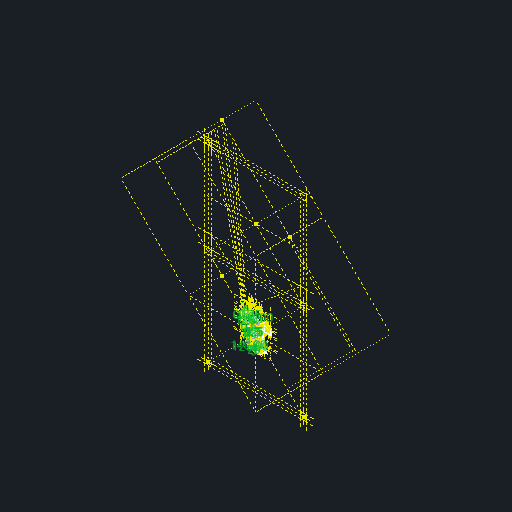
# Autodesk Inventor part: circuit
Saved by Autodesk Inventor 2023.5 (Build 275446000, 446)
## iProperties
Created: 2025-01-11
Part Number: circuit
Material: 一般
Document SubType Name: Modeling
Designer: IshiiLabHonda
Density: 1 g/cm^3
Appearance: 既定
Author: IshiiLabHonda
Autodesk Inventor part; units mm, degrees
ref_plane "YZ Plane" through (0, 0, 0) normal (1, 0, 0) x (0, 1, 0)
ref_plane "XZ Plane" through (0, 0, 0) normal (0, 1, 0) x (-1, 0, 0)
ref_plane "XY Plane" through (0, 0, 0) normal (0, 0, 1) x (1, 0, 0)
derived "chassis.ipt"
sketch "スケッチ1" plane through (0, 0, 0) normal (0, 0, 1) x (1, 0, 0)
  line L0 (0, 0) -> (0, 1) construction
  line L1 (0, 0) -> (1, 0) construction
  line L2 (-90, 90) -> (90, 90) construction
  line L3 (90, 90) -> (90, -90) construction
  line L4 (90, -90) -> (-90, -90) construction
  line L5 (-90, -90) -> (-90, 90) construction
  line L6 (-90, -90) -> (90, 90) construction
  line L7 (-90, 90) -> (90, -90) construction
  line L8 (-84, 96) -> (-84, 84) construction
  line L9 (-84, 84) -> (-96, 84) construction
  line L10 (-96, 84) -> (-96, 96) construction
  line L11 (-96, 96) -> (-84, 84) construction
  line L12 (-84, 96) -> (-96, 84) construction
  line L13 (-96, 96) -> (-84, 96) construction
  line L14 (-96, -96) -> (-96, -84) construction
  line L15 (-84, -96) -> (-96, -96) construction
  line L16 (-96, -96) -> (-84, -84) construction
  line L17 (-96, -84) -> (-84, -96) construction
  line L18 (-84, -84) -> (-84, -96) construction
  line L19 (-96, -84) -> (-84, -84) construction
  line L20 (96, -96) -> (84, -96) construction
  line L21 (96, -84) -> (96, -96) construction
  line L22 (96, -96) -> (84, -84) construction
  line L23 (84, -96) -> (96, -84) construction
  line L24 (84, -84) -> (96, -84) construction
  line L25 (84, -96) -> (84, -84) construction
  line L26 (96, 96) -> (96, 84) construction
  line L27 (84, 96) -> (96, 96) construction
  line L28 (96, 96) -> (84, 84) construction
  line L29 (96, 84) -> (84, 96) construction
  line L30 (84, 84) -> (84, 96) construction
  line L31 (96, 84) -> (84, 84) construction
  line L32 (-84, 84) -> (-84, -84) construction
  line L33 (-96, 84) -> (-96, -84) construction
  line L34 (-84, -84) -> (84, -84) construction
  line L35 (-84, -96) -> (84, -96) construction
  line L36 (96, 84) -> (96, -84) construction
  line L37 (84, 84) -> (84, -84) construction
  line L38 (-84, 96) -> (84, 96) construction
  line L39 (-84, 84) -> (84, 84) construction
  line L40 (-16, 15) -> (16, 15) construction
  line L41 (16, 15) -> (16, -15) construction
  line L42 (16, -15) -> (-16, -15) construction
  line L43 (-16, -15) -> (-16, 15) construction
  line L44 (-16, 15) -> (16, -15) construction
  line L45 (16, 15) -> (-16, -15) construction
  line L46 (-27.25, 11.5) -> (-16, 11.5) construction
  line L47 (-16, -11.5) -> (-27.25, -11.5) construction
  line L48 (-27.25, -11.5) -> (-27.25, 11.5) construction
  line L49 (-27.25, 11.5) -> (-16, -11.5) construction
  line L50 (-16, 11.5) -> (-27.25, -11.5) construction
  line L51 (16, 11.5) -> (27.25, -11.5) construction
  line L52 (16, -11.5) -> (27.25, -11.5) construction
  line L53 (27.25, -11.5) -> (27.25, 11.5) construction
  line L54 (27.25, 11.5) -> (16, 11.5) construction
  line L55 (27.25, 11.5) -> (16, -11.5) construction
  line L56 (-16, -10) -> (16, -10) construction
  line L57 (-16, -12.5) -> (16, -12.5) construction
  line L58 (-16, 12.5) -> (16, 12.5) construction
  line L59 (-16, 10) -> (16, 10) construction
  line L60 (-13.5, -15) -> (-13.5, 15) construction
  line L61 (13.5, -15) -> (13.5, 15) construction
  line L62 (-9.5, -10) -> (-9.5, -15) construction
  line L63 (-13.5, -10) -> (-9.5, -15) construction
  line L64 (-13.5, -15) -> (-9.5, -10) construction
  circle A0 centre (-11.5, -12.5) radius 0.8 construction
  line L65 (9.5, -10) -> (9.5, -15) construction
  line L66 (13.5, -10) -> (9.5, -15) construction
  circle A1 centre (11.5, -12.5) radius 0.8 construction
  line L67 (13.5, -15) -> (9.5, -10) construction
  line L68 (-9.5, 10) -> (-9.5, 15) construction
  line L69 (-13.5, 10) -> (-9.5, 15) construction
  line L70 (-13.5, 15) -> (-9.5, 10) construction
  circle A2 centre (-11.5, 12.5) radius 0.8 construction
  line L71 (9.5, 10) -> (9.5, 15) construction
  line L72 (13.5, 10) -> (9.5, 15) construction
  circle A3 centre (11.5, 12.5) radius 0.8 construction
  line L73 (13.5, 15) -> (9.5, 10) construction
  line L74 (-96, 276) -> (-84, 276) construction
  line L75 (-84, 276) -> (-84, 264) construction
  line L76 (-84, 264) -> (-96, 264) construction
  line L77 (-96, 264) -> (-96, 276) construction
  line L78 (-96, 276) -> (-84, 264) construction
  line L79 (-84, 276) -> (-96, 264) construction
  line L80 (-90, 90) -> (-90, 270) construction
  line L81 (-96, 264) -> (-96, 96) construction
  line L82 (-84, 264) -> (-84, 96) construction
  line L83 (84, 264) -> (84, 96) construction
  line L84 (90, 90) -> (90, 270) construction
  line L85 (96, 264) -> (96, 96) construction
  line L86 (84, 264) -> (96, 264) construction
  line L87 (84, 276) -> (84, 264) construction
  line L88 (96, 276) -> (84, 276) construction
  line L89 (96, 276) -> (84, 264) construction
  line L90 (84, 276) -> (96, 264) construction
  line L91 (96, 264) -> (96, 276) construction
  line L92 (-84, 276) -> (84, 276) construction
  line L93 (-84, 264) -> (84, 264) construction
  line L94 (-90, 270) -> (90, 270) construction
  line L95 (-90, 270) -> (90, 90) construction
  line L96 (-90, 90) -> (90, 270) construction
  circle A4 centre (0, 0) radius 15 construction
  line L97 (-96, 120) -> (96, 120) construction
  line L98 (0, 127.2792) -> (0, -127.2792) construction
  line L99 (-127.2792, 0) -> (127.2792, 0) construction
  line L100 (127.2792, 0) -> (0, -127.2792) construction
  line L101 (0, -127.2792) -> (-127.2792, 0) construction
  line L102 (-127.2792, 0) -> (0, 127.2792) construction
  line L103 (0, 127.2792) -> (127.2792, 0) construction
  line L104 (127.2792, 254.5584) -> (254.5584, 127.2792) construction
  line L105 (254.5584, 127.2792) -> (127.2792, 0) construction
  line L106 (127.2792, 0) -> (0, 127.2792) construction
  line L107 (0, 127.2792) -> (127.2792, 254.5584) construction
  line L108 (-127.2792, 254.5584) -> (0, 127.2792) construction
  line L109 (0, 127.2792) -> (-127.2792, 0) construction
  line L110 (-127.2792, 0) -> (-254.5584, 127.2792) construction
  line L111 (-254.5584, 127.2792) -> (-127.2792, 254.5584) construction
  line L112 (0, 381.8377) -> (127.2792, 254.5584) construction
  line L113 (127.2792, 254.5584) -> (0, 127.2792) construction
  line L114 (0, 127.2792) -> (-127.2792, 254.5584) construction
  line L115 (-127.2792, 254.5584) -> (0, 381.8377) construction
  line L116 (190.9188, 63.6396) -> (63.6396, 190.9188) construction
  line L117 (-190.9188, 190.9188) -> (-63.6396, 63.6396) construction
  line L118 (59.397, -59.397) -> (186.6762, 67.8823) construction
  line L119 (59.397, 186.6762) -> (186.6762, 59.397) construction
  line L120 (63.6396, 190.9188) -> (-63.6396, 318.1981) construction
  line L121 (-186.6762, 186.6762) -> (-59.397, 313.9554) construction
  point P0 (-90, -90)
  point P1 (90, -90)
  point P2 (-21.625, 0)
  point P3 (-84, 120)
  point P4 (84, 120)
  point P5 (0, 0)
sketch "スケッチ5" plane through (0, 0, 0) normal (0, 0, 1) x (1, 0, 0)
  line L0 (0, 0) -> (0, 1) construction
  line L1 (27.25, 11.5) -> (16, 11.5) construction
  line L2 (16, 11.5) -> (27.25, -11.5) construction
  line L3 (27.25, 11.5) -> (16, -11.5) construction
  line L4 (27.25, -11.5) -> (27.25, 11.5) construction
  line L5 (16, -11.5) -> (27.25, -11.5) construction
  line L6 (-90, 90) -> (90, 90) construction
  line L7 (-90, -90) -> (90, 90) construction
  line L8 (-90, 90) -> (90, -90) construction
  line L9 (-84, 84) -> (-84, -84) construction
  line L10 (-96, 84) -> (-96, -84) construction
  line L11 (-90, -90) -> (-90, 90) construction
  line L12 (-84, 84) -> (-96, 84) construction
  line L13 (-96, 84) -> (-96, 96) construction
  line L14 (84, 84) -> (84, -84) construction
  line L15 (90, 90) -> (90, -90) construction
  line L16 (96, 84) -> (84, 84) construction
  line L17 (96, 84) -> (96, -84) construction
  line L18 (90, -90) -> (-90, -90) construction
  line L19 (-84, -84) -> (84, -84) construction
  line L20 (-84, -96) -> (84, -96) construction
  line L21 (-84, -84) -> (-84, -96) construction
  line L22 (-96, -96) -> (-96, -84) construction
  line L23 (-84, -96) -> (-96, -96) construction
  line L24 (-96, -96) -> (-84, -84) construction
  line L25 (-96, -84) -> (-84, -96) construction
  line L26 (-96, -84) -> (-84, -84) construction
  line L27 (0, 0) -> (1, 0) construction
  line L28 (-84, 264) -> (-96, 264) construction
  line L29 (-96, 276) -> (-84, 276) construction
  line L30 (-96, 264) -> (-96, 276) construction
  line L31 (-84, 276) -> (-96, 264) construction
  line L32 (-96, 276) -> (-84, 264) construction
  line L33 (-84, 276) -> (-84, 264) construction
  line L34 (84, -96) -> (84, -84) construction
  line L35 (96, -96) -> (84, -96) construction
  line L36 (96, -84) -> (96, -96) construction
  line L37 (96, -96) -> (84, -84) construction
  line L38 (84, -96) -> (96, -84) construction
  line L39 (84, -84) -> (96, -84) construction
  line L40 (-16, 15) -> (16, 15) construction
  line L41 (16, 15) -> (16, -15) construction
  line L42 (13.5, 15) -> (9.5, 10) construction
  line L43 (9.5, 10) -> (9.5, 15) construction
  line L44 (13.5, 10) -> (9.5, 15) construction
  line L45 (13.5, -15) -> (13.5, 15) construction
  line L46 (-16, 10) -> (16, 10) construction
  line L47 (-16, 12.5) -> (16, 12.5) construction
  circle A0 centre (0, 0) radius 15 construction
  line L48 (-16, -10) -> (16, -10) construction
  line L49 (-16, -12.5) -> (16, -12.5) construction
  line L50 (16, -15) -> (-16, -15) construction
  line L51 (-16, 15) -> (16, -15) construction
  line L52 (16, 15) -> (-16, -15) construction
  line L53 (-13.5, -15) -> (-13.5, 15) construction
  line L54 (-16, -15) -> (-16, 15) construction
  line L55 (-27.25, 11.5) -> (-16, 11.5) construction
  line L56 (-16, -11.5) -> (-27.25, -11.5) construction
  line L57 (-27.25, -11.5) -> (-27.25, 11.5) construction
  line L58 (-27.25, 11.5) -> (-16, -11.5) construction
  line L59 (-16, 11.5) -> (-27.25, -11.5) construction
  line L60 (-9.5, 10) -> (-9.5, 15) construction
  circle A1 centre (-11.5, 12.5) radius 0.8 construction
  line L61 (-13.5, 10) -> (-9.5, 15) construction
  line L62 (-13.5, 15) -> (-9.5, 10) construction
  circle A2 centre (11.5, 12.5) radius 0.8 construction
  line L63 (-84, 96) -> (-96, 84) construction
  line L64 (-96, 96) -> (-84, 96) construction
  line L65 (-84, 96) -> (-84, 84) construction
  line L66 (-96, 96) -> (-84, 84) construction
  line L67 (-96, 264) -> (-96, 96) construction
  line L68 (-84, 264) -> (-84, 96) construction
  line L69 (-84, 96) -> (84, 96) construction
  line L70 (-84, 84) -> (84, 84) construction
  line L71 (84, 84) -> (84, 96) construction
  line L72 (96, 96) -> (96, 84) construction
  line L73 (96, 96) -> (84, 84) construction
  line L74 (96, 84) -> (84, 96) construction
  line L75 (-96, 120) -> (96, 120) construction
  line L76 (84, 96) -> (96, 96) construction
  line L77 (-84, 264) -> (84, 264) construction
  line L78 (84, 264) -> (84, 96) construction
  line L79 (-84, 276) -> (84, 276) construction
  line L80 (96, 264) -> (96, 96) construction
  line L81 (-90, 270) -> (90, 270) construction
  line L82 (-90, 270) -> (90, 90) construction
  line L83 (-90, 90) -> (90, 270) construction
  line L84 (90, 90) -> (90, 270) construction
  line L85 (-90, 90) -> (-90, 270) construction
  line L86 (84, 264) -> (96, 264) construction
  line L87 (96, 276) -> (84, 276) construction
  line L88 (96, 276) -> (84, 264) construction
  line L89 (84, 276) -> (96, 264) construction
  line L90 (96, 264) -> (96, 276) construction
  line L91 (84, 276) -> (84, 264) construction
  circle A3 centre (-11.5, -12.5) radius 0.8 construction
  line L92 (-9.5, -10) -> (-9.5, -15) construction
  line L93 (-13.5, -15) -> (-9.5, -10) construction
  line L94 (9.5, -10) -> (9.5, -15) construction
  circle A4 centre (11.5, -12.5) radius 0.8 construction
  line L95 (13.5, -15) -> (9.5, -10) construction
  line L96 (13.5, -10) -> (9.5, -15) construction
  line L97 (-13.5, -10) -> (-9.5, -15) construction
  line L98 (-11.325, 41.9709) -> (-9.0269, 43.8993) construction
  line L99 (-7.0985, 41.6012) -> (-11.325, 41.9709) construction
  circle A5 centre (-9.2117, 41.7861) radius 0.8 construction
  line L100 (-7.0985, 41.6012) -> (-9.3966, 39.6728) construction
  line L101 (-9.0269, 43.8993) -> (-9.3966, 39.6728) construction
  line L102 (-9.3966, 39.6728) -> (-11.325, 41.9709) construction
  line L103 (-27.25, 31.8718) -> (-28, 31.2425) construction
  line L104 (-11.6044, 45) -> (-27.25, 31.8718) construction
  line L105 (-27.25, 45) -> (-28, 45) construction
  line L106 (-9.0269, 43.8993) -> (-7.0985, 41.6012) construction
  line L107 (-27.25, 45) -> (27.25, 45) construction
  line L108 (-4.4723, 41.194) -> (-9.4516, 37.0158) construction
  line L109 (-9.4516, 37.0158) -> (-13.9511, 42.3782) construction
  line L110 (-8.9719, 46.5563) -> (-4.4723, 41.194) construction
  line L111 (0.8414, 45) -> (-27.25, 21.4285) construction
  line L112 (-0.8414, 45) -> (27.25, 21.4285) construction
  line L113 (-16, 15) -> (16, 15) construction
  line L114 (9.5, 10) -> (9.5, 15) construction
  line L115 (-16, 10) -> (16, 10) construction
  circle A6 centre (-11.5, 12.5) radius 0.8 construction
  line L116 (-9.5, 10) -> (-9.5, 15) construction
  line L117 (-13.5, 10) -> (-9.5, 15) construction
  line L118 (-13.5, 15) -> (-9.5, 10) construction
  line L119 (-16, 12.5) -> (16, 12.5) construction
  line L120 (27.25, 45) -> (28, 45) construction
  line L121 (27.25, 11.5) -> (27.25, 45) construction
  line L122 (-11.0762, 35) -> (11.0762, 35) construction
  line L123 (-27.25, 21.4285) -> (-28, 20.7992) construction
  line L124 (-27.25, 11.5) -> (-27.25, 45) construction
  line L125 (-5.1151, 41.96) -> (-10.0944, 37.7819) construction
  line L126 (-9.2117, 41.7861) -> (-8.6975, 41.1732) construction
  line L127 (-9.2117, 41.7861) -> (-8.5989, 42.3003) construction
  line L128 (-4.4723, 41.194) -> (-13.9511, 42.3782) construction
  line L129 (-8.3291, 45.7902) -> (-13.3084, 41.6121) construction
  line L130 (-13.9511, 42.3782) -> (-8.9719, 46.5563) construction
  line L131 (-8.9719, 46.5563) -> (-9.4516, 37.0158) construction
  line L132 (-27.25, 11.5) -> (-16, 11.5) construction
  line L133 (-27.25, 11.5) -> (-16, -11.5) construction
  line L134 (27.25, 11.5) -> (16, 11.5) construction
  line L135 (27.25, -11.5) -> (27.25, 11.5) construction
  line L136 (16, 11.5) -> (27.25, -11.5) construction
  line L137 (27.25, 11.5) -> (16, -11.5) construction
  line L138 (0, 0) -> (0, 1) construction
  line L139 (0, 0) -> (1, 0) construction
  circle A7 centre (0, 0) radius 7.5 construction
  circle A8 centre (0, 0) radius 15 construction
  line L140 (-13.5, -15) -> (-13.5, 15) construction
  circle A9 centre (11.5, 12.5) radius 0.8 construction
  line L141 (-9.5, -10) -> (-9.5, -15) construction
  line L142 (9.5, -10) -> (9.5, -15) construction
  line L143 (13.5, 10) -> (9.5, 15) construction
  line L144 (-13.5, -15) -> (-9.5, -10) construction
  line L145 (13.5, -10) -> (9.5, -15) construction
  line L146 (13.5, 15) -> (9.5, 10) construction
  line L147 (-16, -12.5) -> (16, -12.5) construction
  line L148 (16, -15) -> (-16, -15) construction
  line L149 (-16, 11.5) -> (-27.25, -11.5) construction
  line L150 (16, -11.5) -> (27.25, -11.5) construction
  line L151 (-16, -11.5) -> (-27.25, -11.5) construction
  line L152 (-27.25, -11.5) -> (-27.25, 11.5) construction
  line L153 (13.5, -15) -> (13.5, 15) construction
  line L154 (16, 15) -> (16, -15) construction
  line L155 (-16, -15) -> (-16, 15) construction
  line L156 (-16, 15) -> (16, -15) construction
  line L157 (16, 15) -> (-16, -15) construction
  line L158 (-28, -8.5) -> (28, -8.5) construction
  line L159 (-28, 8.5) -> (28, 8.5) construction
  line L160 (-28, -31) -> (28, -31) construction
  line L161 (-28, 45) -> (-28, -31) construction
  line L162 (28, 45) -> (28, -31) construction
  line L163 (84, -84) -> (96, -84) construction
  line L164 (84, -96) -> (96, -84) construction
  line L165 (96, -96) -> (84, -84) construction
  line L166 (96, -84) -> (96, -96) construction
  line L167 (96, -96) -> (84, -96) construction
  line L168 (-96, 84) -> (-96, -84) construction
  line L169 (-84, 84) -> (-84, -84) construction
  line L170 (-90, -90) -> (-90, 90) construction
  line L171 (-84, -84) -> (84, -84) construction
  line L172 (-84, -96) -> (84, -96) construction
  line L173 (-90, -90) -> (90, 90) construction
  line L174 (90, -90) -> (-90, -90) construction
  line L175 (-90, 90) -> (90, -90) construction
  line L176 (84, 84) -> (84, -84) construction
  line L177 (90, 90) -> (90, -90) construction
  line L178 (96, 84) -> (96, -84) construction
  line L179 (84, -96) -> (84, -84) construction
  line L180 (-16, -10) -> (16, -10) construction
  circle A10 centre (11.5, -12.5) radius 0.8 construction
  line L181 (13.5, -15) -> (9.5, -10) construction
  line L182 (-13.5, -10) -> (-9.5, -15) construction
  line L183 (-84, -84) -> (-84, -96) construction
  line L184 (-96, -84) -> (-84, -84) construction
  line L185 (-84, -96) -> (-96, -96) construction
  line L186 (-96, -96) -> (-84, -84) construction
  line L187 (-96, -84) -> (-84, -96) construction
  line L188 (-96, -96) -> (-96, -84) construction
  circle A11 centre (-11.5, -12.5) radius 0.8 construction
  line L189 (-96, 96) -> (-84, 96) construction
  line L190 (-84, 96) -> (-84, 84) construction
  line L191 (-84, 96) -> (-96, 84) construction
  line L192 (-96, 96) -> (-84, 84) construction
  line L193 (84, 96) -> (96, 96) construction
  line L194 (96, 84) -> (84, 84) construction
  line L195 (96, 96) -> (96, 84) construction
  line L196 (96, 96) -> (84, 84) construction
  line L197 (96, 84) -> (84, 96) construction
  line L198 (-96, 120) -> (96, 120) construction
  line L199 (-84, 96) -> (84, 96) construction
  line L200 (-90, 90) -> (90, 90) construction
  line L201 (-84, 84) -> (-96, 84) construction
  line L202 (-96, 84) -> (-96, 96) construction
  line L203 (-84, 84) -> (84, 84) construction
  line L204 (84, 120) -> (-27.25, 26.6502) construction
  line L205 (-84, 120) -> (27.25, 26.6502) construction
  line L206 (84, 84) -> (84, 96) construction
  line L207 (-84, 264) -> (-96, 264) construction
  line L208 (-90, 90) -> (-90, 270) construction
  line L209 (-96, 264) -> (-96, 96) construction
  line L210 (-84, 264) -> (-84, 96) construction
  line L211 (96, 264) -> (96, 96) construction
  line L212 (84, 264) -> (84, 96) construction
  line L213 (90, 90) -> (90, 270) construction
  line L214 (-90, 90) -> (90, 270) construction
  line L215 (-90, 270) -> (90, 90) construction
  line L216 (-84, 264) -> (84, 264) construction
  line L217 (-90, 270) -> (90, 270) construction
  line L218 (-96, 264) -> (-96, 276) construction
  line L219 (-96, 276) -> (-84, 276) construction
  line L220 (-96, 276) -> (-84, 264) construction
  line L221 (-84, 276) -> (-96, 264) construction
  line L222 (-84, 276) -> (-84, 264) construction
  line L223 (-84, 276) -> (84, 276) construction
  line L224 (84, 264) -> (96, 264) construction
  line L225 (96, 264) -> (96, 276) construction
  line L226 (96, 276) -> (84, 264) construction
  line L227 (96, 276) -> (84, 276) construction
  line L228 (84, 276) -> (96, 264) construction
  line L229 (84, 276) -> (84, 264) construction
  line L230 (-28, 8.5) -> (-16, 8.5) construction
  line L231 (-28, -8.5) -> (-16, -8.5) construction
  line L232 (-16, 8.5) -> (-16, -8.5) construction
  circle A12 centre (0, 0) radius 7.5 construction
  line L233 (28, -8.5) -> (16, -8.5) construction
  line L234 (16, 8.5) -> (16, -8.5) construction
  line L235 (28, 8.5) -> (16, 8.5) construction
  line L236 (28, 8.5) -> (28, 8.5) projected
  line L237 (-28, -8.5) -> (-9.1203, -31) construction
  line L238 (-9.1203, -31) -> (9.1203, -31) construction
  line L239 (28, -8.5) -> (9.1203, -31) construction
  circle A13 centre (-11.5, 12.5) radius 1.05 construction
  circle A14 centre (11.5, 12.5) radius 1.05 construction
  circle A15 centre (-11.5, -12.5) radius 1.05 construction
  circle A16 centre (11.5, -12.5) radius 1.05 construction
  line L240 (-22.25, 21.5) -> (-22.3613, 22.2922) construction
  line L241 (-22.25, 21.5) -> (-21.4578, 21.6113) construction
  circle A17 centre (-22.25, 21.5) radius 0.8 construction
  line L242 (-20.1223, 24.3236) -> (-19.4264, 19.3723) construction
  line L243 (-24.3777, 18.6764) -> (-25.0736, 23.6277) construction
  line L244 (-20.1223, 24.3236) -> (-24.3777, 18.6764) construction
  line L245 (-25.0736, 23.6277) -> (-20.1223, 24.3236) construction
  line L246 (-19.4264, 19.3723) -> (-24.3777, 18.6764) construction
  line L247 (-25.0736, 23.6277) -> (-19.4264, 19.3723) construction
  line L248 (-25.0736, 23.6277) -> (-24.3777, 18.6764) projected
  line L249 (-20.1223, 24.3236) -> (-15.1709, 25.0195) construction
  line L250 (-15.1709, 25.0195) -> (-14.4751, 20.0681) projected
  line L251 (-14.4751, 20.0681) -> (-19.4264, 19.3723) construction
  line L252 (24.3777, 18.6764) -> (19.4264, 19.3723) construction
  line L253 (14.4751, 20.0681) -> (19.4264, 19.3723) construction
  line L254 (15.1709, 25.0195) -> (14.4751, 20.0681) projected
  line L255 (20.1223, 24.3236) -> (15.1709, 25.0195) construction
  line L256 (20.1223, 24.3236) -> (25.0736, 23.6277) construction
  line L257 (25.0736, 23.6277) -> (24.3777, 18.6764) projected
  line L258 (-25.0736, 23.6277) -> (-15.1709, 25.0195) projected
  line L259 (-14.4751, 20.0681) -> (-15.1709, 25.0195) construction
  line L260 (-14.4751, 20.0681) -> (-24.3777, 18.6764) projected
  line L261 (15.1709, 25.0195) -> (25.0736, 23.6277) projected
  line L262 (24.3777, 18.6764) -> (25.0736, 23.6277) construction
  line L263 (24.3777, 18.6764) -> (14.4751, 20.0681) projected
  line L264 (15.1709, 25.0195) -> (14.4751, 20.0681) construction
  line L265 (-8.558, 47.5563) -> (8.558, 47.5563) construction
  line L266 (-8.558, 47.5563) -> (-8.558, 47.5563) construction
  line L267 (-2.558, 47.5563) -> (0.1895, 46.5563) construction
  line L268 (0.1895, 46.5563) -> (-0.1895, 46.5563) construction
  line L269 (-0.1895, 46.5563) -> (2.558, 47.5563) construction
  line L270 (-3.6267, 42.5563) -> (3.6267, 42.5563) construction
  line L271 (-18.2592, 30.2781) -> (-3.6267, 42.5563) construction
  line L272 (-28, 8.5) -> (-22.1166, 36.1792) construction
  line L273 (-22.1166, 36.1792) -> (-8.558, 47.5563) construction
  line L274 (28, 8.5) -> (22.1166, 36.1792) construction
  line L275 (-18.2592, 30.2781) -> (-20.6565, 19) construction
  line L276 (18.2592, 30.2781) -> (20.6565, 19) construction
  line L277 (-20.6565, 19) -> (20.6565, 19) construction
  line L278 (-14.6308, -20) -> (14.6308, -20) construction
  line L279 (14.6308, -20) -> (8.5077, -26) construction
  line L280 (8.5077, -26) -> (-8.5077, -26) construction
  line L281 (-8.5077, -26) -> (-14.6308, -20) construction
  line L282 (-28, -8.5) -> (-28, -12.5) construction
  line L283 (-28, -12.5) -> (-9.1203, -31) construction
  line L284 (28, -8.5) -> (28, -12.5) construction
  line L285 (28, -12.5) -> (9.1203, -31) construction
  line L286 (-28, 8.5) -> (-28, 26.5) construction
  line L287 (-28, 26.5) -> (-23.3435, 30.4073) construction
  line L288 (28, 26.5) -> (23.3435, 30.4073) construction
  line L289 (28, 8.5) -> (28, 26.5) construction
  line L290 (-5.1203, -31) -> (-3.6203, -29.5) construction
  line L291 (-3.6203, -29.5) -> (3.6203, -29.5) construction
  line L292 (3.6203, -29.5) -> (5.1203, -31) construction
  line L293 (22.1166, 36.1792) -> (8.558, 47.5563) construction
  line L294 (18.2592, 30.2781) -> (3.6267, 42.5563) construction
  line L295 (-20.6565, 19) -> (-21.8255, 13.5) construction
  line L296 (-21.8255, 13.5) -> (-17.8255, 13.5) construction
  line L297 (-17.8255, 13.5) -> (-12.3255, 19) construction
  line L298 (20.6565, 19) -> (21.8255, 13.5) construction
  line L299 (21.8255, 13.5) -> (17.8255, 13.5) construction
  line L300 (17.8255, 13.5) -> (12.3255, 19) construction
  line L301 (-14.6308, -20) -> (-21.2643, -13.5) construction
  line L302 (-21.2643, -13.5) -> (-18.2643, -13.5) construction
  line L303 (-18.2643, -13.5) -> (-8.6308, -20) construction
  line L304 (18.2643, -13.5) -> (8.6308, -20) construction
  line L305 (14.6308, -20) -> (21.2643, -13.5) construction
  line L306 (21.2643, -13.5) -> (18.2643, -13.5) construction
  line L307 (-10.5173, 23.5) -> (-4.5173, 23.5)
  line L308 (-4.5173, 23.5) -> (-2, 26.5)
  line L309 (-2, 26.5) -> (2, 26.5)
  line L310 (2, 26.5) -> (4.5173, 23.5)
  line L311 (4.5173, 23.5) -> (10.5173, 23.5)
  line L312 (0, 0) -> (1, 0) construction
  line L313 (0, 0) -> (0, 1) construction
  line L314 (-27.5, 13) -> (-17, 13)
  line L315 (-17, 13) -> (-17, 17.5)
  line L316 (-17, 17.5) -> (-13, 17.5)
  line L317 (27.5, 13) -> (17, 13)
  line L318 (17, 13) -> (17, 17.5)
  line L319 (17, 17.5) -> (13, 17.5)
  circle A18 centre (0, 0) radius 1.5
  line L320 (-13, 17.5) -> (-13, -18)
  line L321 (13, 17.5) -> (13, -18)
  line L322 (-27.5, 21.1132) -> (-10.5173, 23.5)
  line L323 (27.5, 21.1132) -> (10.5173, 23.5)
  circle A19 centre (-7.1308, -17) radius 0.625 construction
  circle A20 centre (-7.1308, -17) radius 0.8 projected
  circle A21 centre (-7.1308, -17) radius 1.5 projected
  line L324 (-8.6308, -20) -> (-8.6308, -15) construction
  circle A22 centre (7.1308, -17) radius 0.625 construction
  circle A23 centre (7.1308, -17) radius 0.8 projected
  circle A24 centre (7.1308, -17) radius 1.5 projected
  circle A25 centre (-9, 15.5) radius 0.625 construction
  circle A26 centre (-9, 15.5) radius 0.8 projected
  circle A27 centre (-9, 15.5) radius 1.5 projected
  circle A28 centre (9, 15.5) radius 0.625 construction
  circle A29 centre (9, 15.5) radius 0.8 projected
  circle A30 centre (9, 15.5) radius 1.5 projected
  circle A31 centre (-21.1204, 28.8416) radius 0.8 projected
  circle A32 centre (-21.1204, 28.8416) radius 1.5 construction
  circle A33 centre (21.1204, 28.8416) radius 0.8 projected
  circle A34 centre (21.1204, 28.8416) radius 1.5 construction
  circle A35 centre (21.1204, 28.8416) radius 0.475 construction
  line L325 (-10, -28) -> (10, -28)
  line L326 (-13, -18) -> (-18.9172, -18)
  line L327 (-18.9172, -18) -> (-18.9172, -20)
  line L328 (13, -18) -> (18.9172, -18)
  line L329 (18.9172, -18) -> (18.9172, -20)
  line L330 (-12.8008, -24) -> (-15.6008, -23.2498)
  line L331 (-15.6008, -23.2498) -> (-18.9172, -20)
  line L332 (12.8008, -24) -> (15.6008, -23.2498)
  line L333 (15.6008, -23.2498) -> (18.9172, -20)
  line L334 (-27.5, 13) -> (-27.5, 21.1132)
  line L335 (27.5, 13) -> (27.5, 21.1132)
  line L336 (-12.8008, -24) -> (-10, -28)
  line L337 (10, -28) -> (12.8008, -24)
  line L338 (-1.25, 25) -> (1.25, 25)
  line L339 (2, 24.25) -> (2, 24.25)
  line L340 (1.25, 23.5) -> (-1.25, 23.5)
  line L341 (-2, 24.25) -> (-2, 24.25)
  arc A36 (-1.25, 25) -> (-2, 24.25) centre (-1.25, 24.25) ccw
  arc A37 (-2, 24.25) -> (-1.25, 23.5) centre (-1.25, 24.25) ccw
  arc A38 (1.25, 23.5) -> (2, 24.25) centre (1.25, 24.25) ccw
  arc A39 (2, 24.25) -> (1.25, 25) centre (1.25, 24.25) ccw
  line L342 (-27.5, 21.1132) -> (-25.114, 27.5075)
  line L343 (-25.114, 27.5075) -> (-16.2015, 28.7601)
  line L344 (-16.2015, 28.7601) -> (-12.1454, 23.2712)
  line L345 (27.5, 21.1132) -> (25.114, 27.5075)
  line L346 (25.114, 27.5075) -> (16.2015, 28.7601)
  line L347 (16.2015, 28.7601) -> (12.1454, 23.2712)
  line L348 (-26.8721, 25.6471) -> (-13.9987, 27.4563) projected
  line L349 (-13.9987, 27.4563) -> (-12.6765, 18.0488) projected
  line L350 (-12.6765, 18.0488) -> (-25.55, 16.2395) projected
  line L351 (-25.55, 16.2395) -> (-26.8721, 25.6471) projected
  line L352 (-22.1166, 36.1792) -> (-18.2592, 30.2781) construction
  line L353 (-18.8107, 27.6837) -> (-23, 24.1685) construction
  line L354 (-23, 24.1685) -> (-23, 13.5) construction
  line L355 (-21.8255, 13.5) -> (-23, 13.5) construction
  line L356 (18.8107, 27.6837) -> (23, 24.1685) construction
  line L357 (23, 24.1685) -> (23, 13.5) construction
  line L358 (21.8255, 13.5) -> (23, 13.5) construction
  circle A40 centre (-25.5, 18.5) radius 0.8 projected
  circle A41 centre (-25.5, 18.5) radius 1.5 projected
  circle A42 centre (-25.5, 18.5) radius 0.475 construction
  line L359 (-16.2015, 28.7601) -> (-10.5173, 23.5)
  line L360 (16.2015, 28.7601) -> (10.5173, 23.5)
  circle A43 centre (25.5, 18.5) radius 0.475 construction
  circle A44 centre (25.5, 18.5) radius 0.8 projected
  circle A45 centre (25.5, 18.5) radius 1.5 projected
  line L361 (-11.6044, 45) -> (11.6044, 45) projected
  circle A46 centre (-6.875, 0) radius 0.9
  circle A47 centre (-6.875, 0) radius 0.8 construction
  circle A48 centre (6.875, 0) radius 0.9
  circle A49 centre (6.875, 0) radius 0.8 construction
  circle A50 centre (0, 0) radius 5.75 construction
  circle A51 centre (-6.875, 0) radius 0.625 construction
  circle A52 centre (0, 0) radius 4.25
  line L362 (26.8721, 25.6471) -> (13.9987, 27.4563) projected
  line L363 (13.9987, 27.4563) -> (12.6765, 18.0488) projected
  line L364 (12.6765, 18.0488) -> (25.55, 16.2395) projected
  line L365 (25.55, 16.2395) -> (26.8721, 25.6471) projected
  line L366 (-23.5658, 29.3614) -> (-18.675, 28.3218) construction
  line L367 (-20.1879, 33.2287) -> (-25.4441, 8.5) construction
  line L368 (-11.6068, 41.9956) -> (-9.0022, 44.1811) projected
  line L369 (-9.0022, 44.1811) -> (-6.8167, 41.5765) projected
  line L370 (-6.8167, 41.5765) -> (-9.4213, 39.391) projected
  line L371 (-9.4213, 39.391) -> (-11.6068, 41.9956) projected
  line L372 (-11.6068, 41.9956) -> (-6.8167, 41.5765) construction
  line L373 (-9.0022, 44.1811) -> (-9.4213, 39.391) construction
  line L374 (11.6068, 41.9956) -> (9.0022, 44.1811) projected
  line L375 (9.4213, 39.391) -> (11.6068, 41.9956) projected
  line L376 (6.8167, 41.5765) -> (9.4213, 39.391) projected
  line L377 (9.0022, 44.1811) -> (6.8167, 41.5765) projected
  circle A53 centre (-9.2117, 41.7861) radius 1.05 projected
  circle A54 centre (9.2117, 41.7861) radius 1.05 projected
  point P0 (-90, -90)
  point P1 (90, -90)
  point P2 (-21.625, 0)
  point P3 (-6.7221, 43.8751)
  point P4 (-5.3815, 45)
  point P5 (0, 49.5156)
  point P6 (-21.625, 0)
  point P7 (-90, -90)
  point P8 (90, -90)
  point P9 (-5.3815, 45)
  point P10 (5.3815, 45)
  point P11 (11.325, 41.9709)
  point P12 (7.0985, 41.6012)
  point P13 (28.2604, 20.217)
  point P14 (29.75, 18.3552)
  point P15 (-2, 25)
  point P16 (-2, 23.5)
  point P17 (-2, 24.25)
  point P18 (2, 24.25)
  point P19 (12.1454, 23.2712)
  point P20 (20.4797, 27.6588)
  point P21 (29.7346, 22.6965)
  point P22 (-20.4797, 27.6588)
  point P23 (-29.7346, 22.6965)
  point P24 (14.9116, 28.1742)
  point P25 (-14.9116, 28.1742)
  point P26 (-24.8143, 26.7824)
  point P27 (-14.9179, 28.2194)
  point P28 (-26.5811, 23.5759)
  point P29 (-13.7076, 25.3851)
  point P30 (13.88, 26.6117)
  point P31 (26.5811, 23.5759)
  point P32 (24.8143, 26.7824)
  point P33 (14.9179, 28.2194)
  point P34 (-13.88, 26.6117)
  point P35 (-25.7493, 25.8049)
  point P36 (-15.1215, 27.2985)
  point P37 (15.1215, 27.2985)
  point P38 (25.7493, 25.8049)
  point P39 (14.688, 27.3595)
  point P40 (13.7076, 25.3851)
  point P41 (-14.688, 27.3595)
  dimension "d4" = 3
  dimension "d22" = 0.5
  dimension "d23" = 2.5
  dimension "d24" = 3
  dimension "d25" = 1
  dimension "d26" = 2
  dimension "d27" = 3
  dimension "d28" = 125
  dimension "d29" = 140
  dimension "d30" = 20
  dimension "d31" = 4
  dimension "d32" = 4
  dimension "d33" = 1.5
  dimension "d34" = 1.5
  dimension "d35" = 0.75
  dimension "d36" = 6
  dimension "d37" = 130
  dimension "d38" = 4
  dimension "d43" = 6
  dimension "d46" = 4
  dimension "d52" = 9
  dimension "d57" = 1.5
  dimension "d58" = 0.5
  dimension "d61" = 6
  dimension "d75" = 1.6
  dimension "d76" = 0.1
  dimension "d78" = 1.25
  dimension "d79" = 0.5
  dimension "d82" = 1.5
  dimension "d83" = 8.5
  constraints: 80 end point, 20 horizontal alignment, 12 centre point, 12 parallel, 8 point on circle, 8 tangent, 6 coincident, 6 point on line, 5 equal radius, 3 horizontal, 2 symmetric about line, 2 vertical, 1 collinear, 1 perpendicular, 38 other
  measures "d4" diameter of A18
  measures "d22" distance between parallel lines of L53 L320
  measures "d25" distance between parallel lines of L283 L331
  measures "d26" distance of L326.end L327.end
  measures "d27" distance between parallel lines of L238 L325
  measures "d28" angle of L336 L325
  measures "d29" angle of L336 L330
  measures "d30" distance of L325.start L325.end
  measures "d31" distance from line of L330.start L325
  measures "d32" distance of L308.end L309.end
  measures "d33" distance between parallel lines of L338 L309
  measures "d34" distance of point (-2, 23.5) point (-2, 25)
  measures "d35" radius of A36
  measures "d36" distance between parallel lines of L316 L307
  measures "d37" angle of L309 L308
  measures "d38" distance of L339.start L341.end
  measures "d43" distance of L307.start L307.end
  measures "d46" distance of L315.end L316.end
  measures "d52" distance of L342.end L343.end
  measures "d57" distance between parallel lines of L55 L314
  measures "d58" distance between parallel lines of L286 L334
  measures "d61" distance between parallel lines of L322 L343
  measures "d75" diameter of A47
  measures "d76" radial gap between concentric circles of A47 A46
  measures "d78" diameter of A51
  measures "d82" radial gap between concentric circles of A50 A52
  measures "d83" diameter of A52
extrude "押し出し1" add sketch "スケッチ5" against normal blind 0.8 contours L322 L250 L260 A41 L248 | L248 A41 L351 L322 | A41 L260 L248 | L248 L260 A41 L351 A40 | L351 A41 L350 L315 L314 L334 L322 | L322 L349 L350 L316 L315 L351 A41 L260 L250 | L351 A40 A41 | L322 L307 L308 L309 L310 L311 L323 L363 L364 L319 L321 L328 L329 L333 L332 L337 L325 L336 L330 L331 L327 L326 L320 L316 L350 L349 | A40 L351 | L351 A40 | L323 L254 L263 A45 L365 L364 L318 L319 L363 | L323 L257 A45 L263 L254 | L323 L365 A45 L257 | A45 L257 L263 | L263 L257 A45 L365 A44 | L323 L335 L317 L318 L364 L365 A45 | L365 A44 A45 | L365 A44 | A44 L365 | A18 | A20 | A21 | A23 | A24 | A26 | A27 | A29 | A30 | L338 A39 A38 L340 A37 A36 | A46 | A48 | A52
extrude "押し出し5" cut sketch "スケッチ5" against normal blind 0.8 contours A20 | A23 | A26 | A29
extrude "押し出し8" add sketch "スケッチ5" against normal blind 0.8 contours L322 L250 L260 A41 L248 | L248 A41 L351 L322 | A41 L260 L248 | L248 L260 A41 L351 A40 | L351 A41 L350 L315 L314 L334 L322 | L322 L349 L350 L316 L315 L351 A41 L260 L250 | L351 A40 A41 | L322 L307 L308 L309 L310 L311 L323 L363 L364 L319 L321 L328 L329 L333 L332 L337 L325 L336 L330 L331 L327 L326 L320 L316 L350 L349 | A40 L351 | L351 A40 | L323 L254 L263 A45 L365 L364 L318 L319 L363 | L323 L257 A45 L263 L254 | L323 L365 A45 L257 | A45 L257 L263 | L263 L257 A45 L365 A44 | L323 L335 L317 L318 L364 L365 A45 | L365 A44 A45 | L365 A44 | A44 L365 | A18 | A20 | A21 | A23 | A24 | A26 | A27 | A29 | A30 | L338 A39 A38 L340 A37 A36 | A46 | A48 | A52
extrude "押し出し10" cut sketch "スケッチ5" against normal blind 0.8 contours A20 | A23 | A26 | A29 | L338 A39 A38 L340 A37 A36
extrude "押し出し12" add sketch "スケッチ5" against normal blind 0.8 contours L258 L250 L322 L248 | L248 L322 L351 L342 L348 L344 L349 L250 L258 | L322 L342 L351 | L349 L344 L322 | L342 L343 A31 L344 L348 | L343 A31 | L347 L363 L323 | L363 L347 L362 L345 L365 L323 L257 L261 L254 | L254 L261 L257 L323 | L347 L346 A33 L345 L362 | L346 A33 | L365 L345 L323 picked at (-21.0384, 28.0699) picked at (21.0384, 28.0699)
extrude "押し出し14" cut sketch "スケッチ5" against normal blind 1 contours A40 L351 | L351 A40
extrude "押し出し15" add sketch "スケッチ5" against normal blind 0.8 contours L344 L349 L359 L322 | L344 L348 L359 L349 | L344 L359 L348 | L360 L363 L347 L323 | L360 L362 L347 L363 | L360 L347 L362
extrude "押し出し16" cut sketch "スケッチ5" against normal blind 0.8 contours L365 A44 | A44 L365
extrude "押し出し17" [suppressed]
chamfer "面取り1" distance 0.8 angle 45 4 edges at (-17, 17.5, -0.4) (-13, 17.5, -0.4) (13, 17.5, -0.4) (17, 17.5, -0.4)
chamfer "面取り2" distance 0.8 angle 45 4 edges at (-17, 13, -0.4) (-27.5, 13, -0.4) (17, 13, -0.4) (27.5, 13, -0.4)
mirror "ミラー1" [suppressed]
extrude "押し出し18" cut sketch "スケッチ5" against normal blind 5 contours A18 | A46 | A48
extrude "押し出し19" cut sketch "スケッチ5" against normal blind 0.2 contours L258 L250 L322 L248 | L248 L322 L351 L342 L348 L344 L349 L250 L258 | L322 L250 L260 A41 L248 | L248 A41 L351 L322 | A41 L260 L248 | L248 L260 A41 L351 A40 | L322 L349 L350 L316 L315 L351 A41 L260 L250 | L351 L348 L342 | A40 L351 | L342 L343 A31 L344 L348 | L344 L348 L359 L349 | L344 L359 L348 | L359 L348 L349 | L350 L315 L316 | L343 A31 | L363 L362 L360 | L360 L362 L347 L363 | L363 L347 L362 L345 L365 L323 L257 L261 L254 | L323 L254 L263 A45 L365 L364 L318 L319 L363 | L360 L347 L362 | L323 L257 A45 L263 L254 | L254 L261 L257 L323 | L347 L346 A33 L345 L362 | L323 L365 A45 L257 | L319 L318 L364 | L362 L365 L345 | L346 A33 | A45 L257 L263 | L263 L257 A45 L365 A44 | A44 L365 picked at (-25.1094, 18.423) picked at (-21.0384, 28.0699) picked at (21.0384, 28.0699) picked at (25.4802, 18.4078)
chamfer "面取り3" distance 1 angle 45 2 edges at (-13, -18, -0.4) (13, -18, -0.4)
sketch "スケッチ4" plane through (0, 0, 0) normal (0, 0, 1) x (1, 0, 0)
  line L0 (-84, 264) -> (-96, 264) construction
  line L1 (-90, 90) -> (-90, 270) construction
  line L2 (-96, 264) -> (-96, 96) construction
  line L3 (-96, 96) -> (-84, 96) construction
  line L4 (-84, 96) -> (-84, 84) construction
  line L5 (-84, 96) -> (-96, 84) construction
  line L6 (-96, 96) -> (-84, 84) construction
  line L7 (-84, 264) -> (-84, 96) construction
  line L8 (-84, 84) -> (-96, 84) construction
  line L9 (84, -84) -> (96, -84) construction
  line L10 (84, -96) -> (96, -84) construction
  line L11 (96, -96) -> (84, -84) construction
  line L12 (96, -84) -> (96, -96) construction
  line L13 (96, -96) -> (84, -96) construction
  line L14 (0, 0) -> (0, 1) construction
  line L15 (0, 0) -> (1, 0) construction
  line L16 (13.5, 15) -> (9.5, 10) construction
  line L17 (-96, 84) -> (-96, -84) construction
  line L18 (-84, 84) -> (-84, -84) construction
  line L19 (-90, -90) -> (-90, 90) construction
  line L20 (-90, 90) -> (90, 90) construction
  line L21 (-84, -84) -> (84, -84) construction
  line L22 (-84, -96) -> (84, -96) construction
  line L23 (-90, -90) -> (90, 90) construction
  line L24 (90, -90) -> (-90, -90) construction
  line L25 (-90, 90) -> (90, -90) construction
  line L26 (84, 84) -> (84, -84) construction
  line L27 (90, 90) -> (90, -90) construction
  line L28 (96, 84) -> (96, -84) construction
  line L29 (-96, 84) -> (-96, 96) construction
  line L30 (-84, -84) -> (-84, -96) construction
  line L31 (-96, -84) -> (-84, -84) construction
  line L32 (-84, -96) -> (-96, -96) construction
  line L33 (-96, -96) -> (-84, -84) construction
  line L34 (-96, -84) -> (-84, -96) construction
  line L35 (-96, -96) -> (-96, -84) construction
  line L36 (84, -96) -> (84, -84) construction
  line L37 (-16, -15) -> (-16, 15) construction
  line L38 (-27.25, 11.5) -> (-16, 11.5) construction
  line L39 (-16, -11.5) -> (-27.25, -11.5) construction
  line L40 (-16, 11.5) -> (-27.25, -11.5) construction
  line L41 (-27.25, 11.5) -> (-16, -11.5) construction
  line L42 (-27.25, -11.5) -> (-27.25, 11.5) construction
  line L43 (9.5, 10) -> (9.5, 15) construction
  circle A0 centre (11.5, 12.5) radius 0.8 construction
  line L44 (27.25, 11.5) -> (16, 11.5) construction
  line L45 (13.5, 10) -> (9.5, 15) construction
  circle A1 centre (11.5, -12.5) radius 0.8 construction
  line L46 (13.5, -15) -> (9.5, -10) construction
  line L47 (13.5, -10) -> (9.5, -15) construction
  line L48 (9.5, -10) -> (9.5, -15) construction
  circle A2 centre (-11.5, -12.5) radius 0.8 construction
  line L49 (-9.5, -10) -> (-9.5, -15) construction
  line L50 (-13.5, -15) -> (-9.5, -10) construction
  line L51 (-13.5, -10) -> (-9.5, -15) construction
  line L52 (96, 84) -> (84, 84) construction
  line L53 (96, 96) -> (96, 84) construction
  line L54 (84, 96) -> (96, 96) construction
  line L55 (96, 96) -> (84, 84) construction
  line L56 (84, 84) -> (84, 96) construction
  line L57 (96, 84) -> (84, 96) construction
  line L58 (-96, 264) -> (-96, 276) construction
  line L59 (-84, 276) -> (-84, 264) construction
  line L60 (-96, 276) -> (-84, 276) construction
  line L61 (-96, 276) -> (-84, 264) construction
  line L62 (-84, 276) -> (-96, 264) construction
  line L63 (-84, 84) -> (84, 84) construction
  line L64 (-84, 96) -> (84, 96) construction
  line L65 (84, 264) -> (84, 96) construction
  line L66 (90, 90) -> (90, 270) construction
  line L67 (-90, 90) -> (90, 270) construction
  line L68 (-90, 270) -> (90, 90) construction
  line L69 (96, 264) -> (96, 96) construction
  line L70 (-96, 120) -> (96, 120) construction
  line L71 (-84, 264) -> (84, 264) construction
  line L72 (-84, 276) -> (84, 276) construction
  line L73 (-90, 270) -> (90, 270) construction
  line L74 (84, 276) -> (84, 264) construction
  line L75 (84, 264) -> (96, 264) construction
  line L76 (96, 264) -> (96, 276) construction
  line L77 (96, 276) -> (84, 264) construction
  line L78 (96, 276) -> (84, 276) construction
  line L79 (84, 276) -> (96, 264) construction
  line L80 (-16, 15) -> (16, 15) construction
  line L81 (16, 15) -> (16, -15) construction
  line L82 (16, -15) -> (-16, -15) construction
  circle A3 centre (-11.5, 12.5) radius 0.8 construction
  line L83 (-13.5, 10) -> (-9.5, 15) construction
  line L84 (-9.5, 10) -> (-9.5, 15) construction
  line L85 (-13.5, 15) -> (-9.5, 10) construction
  circle A4 centre (0, 0) radius 15 construction
  line L86 (-16, 10) -> (16, 10) construction
  line L87 (-16, 12.5) -> (16, 12.5) construction
  line L88 (-16, 15) -> (16, -15) construction
  line L89 (16, 15) -> (-16, -15) construction
  line L90 (-16, -10) -> (16, -10) construction
  line L91 (-16, -12.5) -> (16, -12.5) construction
  line L92 (13.5, -15) -> (13.5, 15) construction
  line L93 (16, 11.5) -> (27.25, -11.5) construction
  line L94 (16, -11.5) -> (27.25, -11.5) construction
  line L95 (27.25, -11.5) -> (27.25, 11.5) construction
  line L96 (27.25, 11.5) -> (16, -11.5) construction
  line L97 (-13.5, -15) -> (-13.5, 15) construction
  line L98 (-84, 120) -> (27.25, 26.6502) construction
  line L99 (84, 120) -> (-27.25, 26.6502) construction
  line L100 (-27.25, 45) -> (27.25, 45) construction
  line L101 (0.8414, 45) -> (-27.25, 21.4285) construction
  line L102 (-0.8414, 45) -> (27.25, 21.4285) construction
  line L103 (-11.6044, 45) -> (-27.25, 31.8718) construction
  line L104 (-8.9719, 46.5563) -> (-4.4723, 41.194) construction
  line L105 (-4.4723, 41.194) -> (-9.4516, 37.0158) construction
  line L106 (-9.4516, 37.0158) -> (-13.9511, 42.3782) construction
  line L107 (-13.9511, 42.3782) -> (-8.9719, 46.5563) construction
  line L108 (-8.9719, 46.5563) -> (-9.4516, 37.0158) construction
  line L109 (-4.4723, 41.194) -> (-13.9511, 42.3782) construction
  line L110 (-8.3291, 45.7902) -> (-13.3084, 41.6121) construction
  line L111 (-5.1151, 41.96) -> (-10.0944, 37.7819) construction
  line L112 (-9.2117, 41.7861) -> (-8.5989, 42.3003) construction
  line L113 (-9.2117, 41.7861) -> (-8.6975, 41.1732) construction
  line L114 (-9.0269, 43.8993) -> (-7.0985, 41.6012) construction
  line L115 (-7.0985, 41.6012) -> (-9.3966, 39.6728) construction
  line L116 (-9.3966, 39.6728) -> (-11.325, 41.9709) construction
  line L117 (-11.325, 41.9709) -> (-9.0269, 43.8993) construction
  line L118 (-9.0269, 43.8993) -> (-9.3966, 39.6728) construction
  line L119 (-7.0985, 41.6012) -> (-11.325, 41.9709) construction
  circle A5 centre (-9.2117, 41.7861) radius 0.8 construction
  line L120 (-27.25, 11.5) -> (-27.25, 45) construction
  line L121 (27.25, 11.5) -> (27.25, 45) construction
  line L122 (-11.0762, 35) -> (11.0762, 35) construction
  line L123 (-28, 45) -> (-28, -31) construction
  line L124 (28, 45) -> (28, -31) construction
  line L125 (-27.25, 45) -> (-28, 45) construction
  line L126 (27.25, 45) -> (28, 45) construction
  line L127 (-28, 8.5) -> (28, 8.5) construction
  line L128 (-28, -8.5) -> (28, -8.5) construction
  circle A6 centre (0, 0) radius 7.5 construction
  line L129 (-28, -31) -> (28, -31) construction
  line L130 (-27.25, 31.8718) -> (-28, 31.2425) construction
  line L131 (-27.25, 21.4285) -> (-28, 20.7992) construction
  line L132 (-22.25, 21.5) -> (-22.3613, 22.2922) construction
  line L133 (-22.25, 21.5) -> (-21.4578, 21.6113) construction
  line L134 (-25.0736, 23.6277) -> (-20.1223, 24.3236) construction
  line L135 (-20.1223, 24.3236) -> (-19.4264, 19.3723) construction
  line L136 (-19.4264, 19.3723) -> (-24.3777, 18.6764) construction
  line L137 (-24.3777, 18.6764) -> (-25.0736, 23.6277) construction
  line L138 (-25.0736, 23.6277) -> (-19.4264, 19.3723) construction
  line L139 (-20.1223, 24.3236) -> (-24.3777, 18.6764) construction
  circle A7 centre (-22.25, 21.5) radius 0.8 construction
  line L140 (-22.25, 45) -> (-22.25, -31) construction
  line L141 (-96, 180) -> (96, 180) construction
  line L142 (-22.3613, 22.2922) -> (-62.8646, 310.4878) construction
  line L143 (-186.6762, 186.6762) -> (-59.397, 313.9554) construction
  line L144 (59.397, 186.6762) -> (186.6762, 59.397) construction
  line L145 (-22.25, 21.5) -> (-77.9717, 295.3807) construction
  line L146 (-22.25, 21.5) -> (-44.0597, 298.6181) construction
  line L147 (63.6396, 190.9188) -> (-63.6396, 318.1981) construction
  line L148 (9.2117, 41.7861) -> (8.5989, 42.3003) construction
  line L149 (9.2117, 41.7861) -> (8.6975, 41.1732) construction
  circle A8 centre (9.2117, 41.7861) radius 0.8 construction
  line L150 (11.325, 41.9709) -> (9.0269, 43.8993) construction
  line L151 (9.0269, 43.8993) -> (9.3966, 39.6728) construction
  line L152 (9.3966, 39.6728) -> (11.325, 41.9709) construction
  line L153 (9.4516, 37.0158) -> (13.9511, 42.3782) construction
  line L154 (7.0985, 41.6012) -> (9.3966, 39.6728) construction
  line L155 (5.1151, 41.96) -> (10.0944, 37.7819) construction
  line L156 (9.0269, 43.8993) -> (7.0985, 41.6012) construction
  line L157 (4.4723, 41.194) -> (13.9511, 42.3782) construction
  line L158 (8.3291, 45.7902) -> (13.3084, 41.6121) construction
  line L159 (7.0985, 41.6012) -> (11.325, 41.9709) construction
  line L160 (4.4723, 41.194) -> (9.4516, 37.0158) construction
  line L161 (8.9719, 46.5563) -> (4.4723, 41.194) construction
  line L162 (13.9511, 42.3782) -> (8.9719, 46.5563) construction
  line L163 (8.9719, 46.5563) -> (9.4516, 37.0158) construction
  line L164 (-20.1223, 24.3236) -> (-15.1709, 25.0195) construction
  line L165 (-15.1709, 25.0195) -> (-14.4751, 20.0681) construction
  line L166 (-14.4751, 20.0681) -> (-19.4264, 19.3723) construction
  line L167 (-20.1223, 24.3236) -> (-25.0736, 23.6277) construction
  line L168 (-25.0736, 23.6277) -> (-24.3777, 18.6764) construction
  line L169 (-24.3777, 18.6764) -> (-19.4264, 19.3723) construction
  line L170 (20.1223, 24.3236) -> (25.0736, 23.6277) construction
  line L171 (24.3777, 18.6764) -> (19.4264, 19.3723) construction
  line L172 (14.4751, 20.0681) -> (19.4264, 19.3723) construction
  line L173 (24.3777, 18.6764) -> (25.0736, 23.6277) construction
  line L174 (15.1709, 25.0195) -> (14.4751, 20.0681) construction
  line L175 (20.1223, 24.3236) -> (15.1709, 25.0195) construction
  line L176 (25.0736, 23.6277) -> (24.3777, 18.6764) construction
  line L177 (20.1223, 24.3236) -> (24.3777, 18.6764) construction
  line L178 (19.4264, 19.3723) -> (25.0736, 23.6277) construction
  line L179 (-17.2987, 22.1959) -> (-58.4376, 314.9148) construction
  line L180 (-17.2987, 22.1959) -> (-38.6259, 293.1844) construction
  line L181 (-17.2987, 22.1959) -> (-73.7397, 299.6126) construction
  line L182 (-20.1223, 24.3236) -> (-14.4751, 20.0681) construction
  line L183 (-19.4264, 19.3723) -> (-15.1709, 25.0195) construction
  line L184 (-13.9511, 42.3782) -> (-16.2493, 40.4498) construction
  line L185 (-16.2493, 40.4498) -> (-11.7498, 35.0875) construction
  line L186 (-11.7498, 35.0875) -> (-9.4516, 37.0158) construction
  point P0 (90, -90)
  point P1 (-90, -90)
  point P2 (-21.625, 0)
  point P3 (0, 49.5156)
  point P4 (-5.3815, 45)
  point P5 (-6.7221, 43.8751)
  point P6 (0, 180)
  point P7 (6.7221, 43.8751)
  constraints: 2 other
